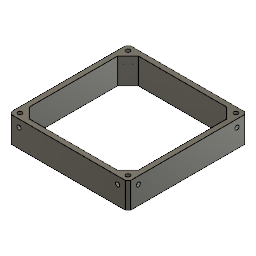
stucture lower fossasat v2 (Autodesk Fusion 360 design; units mm, degrees)
Autodesk Fusion 360 part; units mm, degrees
note: some values were not read from the file. Set by a fixed rule: which sketch regions a step uses.
sketch "Sketch1" plane through (0, 0, 0) normal (0, 1, 0) x (1, 0, 0)
  line L0 (0, 0) -> (46, 0)
  line L1 (46, 0) -> (46, -46)
  line L2 (46, -46) -> (0, -46)
  line L3 (0, -46) -> (0, 0)
  line L4 (0, 0) -> (6.364, -6.364)
  line L5 (0, 0) -> (9, 0) construction
  line L6 (6.364, -6.364) -> (0, -6.364)
  line L7 (0, -6.364) -> (0, 0)
  line L8 (0, 0) -> (6.364, 0)
  line L9 (6.364, 0) -> (6.364, -6.364)
  line L10 (46, -46) -> (37, -46)
  line L11 (37, -46) -> (37, -37)
  line L12 (37, -37) -> (46, -37)
  line L13 (46, -37) -> (46, -46)
  line L14 (46, 0) -> (37, 0)
  line L15 (37, 0) -> (37, -9)
  line L16 (37, -9) -> (46, -9)
  line L17 (46, -9) -> (46, 0)
  line L18 (0, -46) -> (9, -46)
  line L19 (9, -46) -> (9, -37)
  line L20 (9, -37) -> (0, -37)
  line L21 (0, -37) -> (0, -46)
  line L22 (0, -46) -> (2, -46)
  line L23 (2, -46) -> (2, -44)
  circle A0 centre (2, -44) radius 1
  circle A1 centre (2, -44) radius 0.8
  line L24 (23, 0) -> (23, -46)
  line L25 (23, -23) -> (42, -23)
  line L26 (42, -23) -> (42, -42)
  line L27 (42, -42) -> (4, -42)
  line L28 (4, -42) -> (4, -4)
  line L29 (4, -4) -> (42, -4)
  line L30 (42, -4) -> (42, -42)
  line L31 (4, -42) -> (8, -46)
  line L32 (4, -42) -> (9.6569, -42) construction
  line L33 (8, -46) -> (0, -38)
  line L34 (46, -46) -> (44, -46)
  line L35 (44, -46) -> (44, -44)
  circle A2 centre (44, -44) radius 0.8
  line L36 (42, -42) -> (46, -38)
  line L37 (42, -42) -> (38, -46)
  line L38 (46, 0) -> (44, 0)
  line L39 (44, 0) -> (44, -2)
  circle A3 centre (44, -2) radius 0.8
  line L40 (42, -4) -> (46, -8)
  line L41 (46, -8) -> (38, 0)
  line L42 (4, -4) -> (8, 0)
  line L43 (4, -4) -> (0, -8)
  line L44 (0, 0) -> (1.4142, -1.4142)
  circle A4 centre (1.4142, -1.4142) radius 0.8
  line L45 (23, 0) -> (23, -2)
  line L46 (40, -2) -> (6, -2)
  line L47 (44, -6) -> (44, -40)
  line L48 (40, -44) -> (6, -44)
  line L49 (2, -40) -> (2, -6)
  dimension "d1" = 46
  dimension "d2" = 46
  dimension "d3" = 45
  dimension "d4" = 9
  dimension "d5" = 9
  dimension "d6" = 9
  dimension "d7" = 9
  dimension "d8" = 9
  dimension "d9" = 9
  dimension "d10" = 2
  dimension "d11" = 1.6
  dimension "d12" = 19
  dimension "d13" = 19
  dimension "d14" = 45
  dimension "d15" = 1.6
  measures "d3" angle of L4 L5
  measures "d4" distance of L0.start
  measures "d8" distance of L0.start
  measures "d10" distance of L0.start
  measures "d11" diameter of A1
  measures "d14" angle of L31 L32
  measures "d15" diameter of A2
extrude "Extrude1" add sketch "Sketch1" along normal blind 10 contours L3 L4 L6 L7 L43 L44 A4 | L0 L4 L8 L9 L42 L44 A4 | L0 L9 L42 | L3 L6 L43 | L0 L9 L24 L42 L45 L46 | L9 L42 L46 | L3 L6 L20 L43 L49 | L0 L15 L24 L45 L46 | L3 L20 L21 L33 L49 | L0 L14 L15 L41 L46 | L2 L3 L18 L21 L22 L31 L33 | L0 L1 L14 L17 L38 L40 L41 | L2 L18 L19 L31 L33 L48 | L1 L16 L17 L40 L41 L47 | L2 L11 L24 L48 | L2 L19 L24 L48 | L1 L12 L16 L47 | L2 L10 L11 L37 L48 | L1 L2 L10 L13 L34 L36 L37 | L1 L12 L13 L36 L47
sketch "Sketch2" plane through (46, 0, 0) normal (1, 0, 0) x (0, 0, -1)
  line L0 (-46, 0) -> (0, 0)
  line L1 (0, 0) -> (0, 10)
  line L2 (0, 10) -> (-46, 10)
  line L3 (-46, 10) -> (-46, 0)
  line L4 (-43, 0) -> (-43, 7.15)
  line L5 (-43, 7.15) -> (-46.6287, 7.15)
  line L6 (-46, 7.15) -> (-42, 7.15)
  circle A0 centre (-42, 7.15) radius 0.8
extrude "Extrude2" cut sketch "Sketch2" against normal blind 3 contours A0
sketch "Sketch3" plane through (0, 0, 46) normal (0, 0, 1) x (1, 0, 0)
  line L0 (0, 0) -> (46, 0)
  line L1 (46, 0) -> (46, 10)
  line L2 (46, 10) -> (0, 10)
  line L3 (0, 10) -> (0, 0)
  line L4 (43.2, 0) -> (43.2, 7.15)
  line L5 (43.2, 7.15) -> (46.5827, 7.15)
  line L6 (46, 7.15) -> (42, 7.15)
  circle A0 centre (42, 7.15) radius 0.8
  dimension "d20" = 7.15
  dimension "d21" = 1.6
  measures "d20" distance of L0.start
  measures "d21" diameter of A0
extrude "Extrude3" cut sketch "Sketch3" against normal blind 3 contours A0
sketch "Sketch4" plane through (46, 0, 0) normal (1, 0, 0) x (0, 0, -1)
  circle A0 centre (-42, 7.15) radius 0.8
  line L0 (-46, 0) -> (0, 0)
  line L1 (0, 0) -> (0, 10)
  line L2 (0, 10) -> (-46, 10)
  line L3 (-46, 10) -> (-46, 0)
  line L4 (0, 0) -> (-4, 0)
  line L5 (-4, 0) -> (-4, 7.15)
  circle A1 centre (-4, 7.15) radius 0.8
extrude "Extrude4" cut sketch "Sketch4" against normal blind 3 contours A1
sketch "Sketch5" plane through (0, 0, 0) normal (0, 0, -1) x (-1, 0, 0)
  line L0 (-46, 0) -> (0, 0)
  line L1 (0, 0) -> (0, 10)
  line L2 (0, 10) -> (-46, 10)
  line L3 (-46, 10) -> (-46, 0)
  line L4 (-46, 0) -> (-42, 0)
  line L5 (-42, 0) -> (-42, 7.15)
  circle A0 centre (-42, 7.15) radius 0.8
extrude "Extrude5" cut sketch "Sketch5" against normal blind 3 contours A0
sketch "Sketch6" plane through (0, 0, 0) normal (0, 0, -1) x (-1, 0, 0)
  circle A0 centre (-42, 7.15) radius 0.8
  line L0 (-46, 0) -> (0, 0)
  line L1 (0, 0) -> (0, 10)
  line L2 (0, 10) -> (-46, 10)
  line L3 (-46, 10) -> (-46, 0)
  line L4 (0, 0) -> (-4, 0)
  line L5 (-4, 0) -> (-4, 7.15)
  circle A1 centre (-4, 7.15) radius 0.8
extrude "Extrude6" cut sketch "Sketch6" against normal blind 3 contours A1
sketch "Sketch7" plane through (0, 0, 0) normal (-1, 0, 0) x (0, 0, 1)
  line L0 (0, 0) -> (46, 0)
  line L1 (46, 0) -> (46, 10)
  line L2 (46, 10) -> (0, 10)
  line L3 (0, 10) -> (0, 0)
  line L4 (0, 0) -> (4, 0)
  line L5 (4, 0) -> (4, 7.15)
  line L6 (46, 0) -> (42, 0)
  line L7 (42, 0) -> (42, 7.15)
  circle A0 centre (42, 7.15) radius 0.8
  circle A1 centre (4, 7.15) radius 0.8
extrude "Extrude7" cut sketch "Sketch7" against normal blind 3 contours A0 | A1
sketch "Sketch8" plane through (0, 10, 0) normal (0, 1, 0) x (-1, 0, 0)
  circle A0 centre (-1.4142, 1.4142) radius 0.8
  circle A1 centre (-44, 2) radius 0.8
  line L0 (-44, 40) -> (-42, 42)
  line L1 (-42, 42) -> (-40, 44)
  line L2 (-40, 44) -> (-6, 44)
  line L3 (-6, 44) -> (-2, 40)
  line L4 (-2, 40) -> (-2, 6.364)
  line L5 (-2, 6.364) -> (-1.636, 6.364)
  line L6 (-1.636, 6.364) -> (-6, 2)
  line L7 (-6, 2) -> (-40, 2)
  line L8 (-40, 2) -> (-44, 6)
  line L9 (-44, 6) -> (-44, 40)
  circle A2 centre (-44, 44) radius 0.8
  circle A3 centre (-2, 44) radius 1
  line L10 (-46, 46) -> (-46, 0)
  line L11 (-46, 0) -> (0, 0)
  line L12 (0, 0) -> (0, 46)
  line L13 (0, 46) -> (-46, 46)
  circle A4 centre (-2, 44) radius 1
  circle A5 centre (-2, 44) radius 0.8
extrude "Extrude8" add sketch "Sketch8" against normal blind 10 contours A3 A4
sketch "Sketch9" plane through (0, 0, 46) normal (0, 0, 1) x (1, 0, 0)
  circle A0 centre (42, 7.15) radius 0.8
  line L0 (0, 0) -> (46, 0)
  line L1 (46, 0) -> (46, 10)
  line L2 (46, 10) -> (0, 10)
  line L3 (0, 10) -> (0, 0)
  line L4 (0, 0) -> (4, 0)
  line L5 (4, 0) -> (4, 7.15)
  circle A1 centre (4, 7.15) radius 0.8
extrude "Extrude9" cut sketch "Sketch9" against normal blind 3 contours A1
sketch "Sketch10" plane through (0, 10, 0) normal (0, 1, 0) x (-1, 0, 0)
  circle A0 centre (-2, 44) radius 0.8
  circle A1 centre (-1.4142, 1.4142) radius 0.8
  circle A2 centre (-44, 2) radius 0.8
  line L0 (-44, 40) -> (-42, 42)
  line L1 (-42, 42) -> (-40, 44)
  line L2 (-40, 44) -> (-6, 44)
  line L3 (-6, 44) -> (-2, 40)
  line L4 (-2, 40) -> (-2, 6.364)
  line L5 (-2, 6.364) -> (-1.636, 6.364)
  line L6 (-1.636, 6.364) -> (-6, 2)
  line L7 (-6, 2) -> (-40, 2)
  line L8 (-40, 2) -> (-44, 6)
  line L9 (-44, 6) -> (-44, 40)
  circle A3 centre (-44, 44) radius 0.8
  line L10 (-46, 46) -> (-46, 0)
  line L11 (-46, 0) -> (0, 0)
  line L12 (0, 0) -> (0, 46)
  line L13 (0, 46) -> (-46, 46)
  line L14 (-2, 6.364) -> (-2, 5.5)
  line L15 (-2, 5.5) -> (-1.568, 5.932)
  line L16 (-1.568, 5.932) -> (-1.5, 7)
  line L17 (-1.5, 7) -> (-2, 6.364)
extrude "Extrude10" add sketch "Sketch10" against normal blind 10 contours L5 L6 L14
sketch "Sketch11" plane through (0, 10, 0) normal (0, 1, 0) x (-1, 0, 0)
  circle A0 centre (-2, 44) radius 0.8
  circle A1 centre (-1.4142, 1.4142) radius 0.8
  circle A2 centre (-44, 2) radius 0.8
  line L0 (-44, 40) -> (-42, 42)
  line L1 (-42, 42) -> (-40, 44)
  line L2 (-40, 44) -> (-6, 44)
  line L3 (-6, 44) -> (-2, 40)
  line L4 (-2, 40) -> (-2, 6)
  line L5 (-2, 6) -> (-6, 2)
  line L6 (-6, 2) -> (-40, 2)
  line L7 (-40, 2) -> (-44, 6)
  line L8 (-44, 6) -> (-44, 40)
  circle A3 centre (-44, 44) radius 0.8
  line L9 (-46, 46) -> (-46, 0)
  line L10 (-46, 0) -> (0, 0)
  line L11 (0, 0) -> (0, 46)
  line L12 (0, 46) -> (-46, 46)
  circle A4 centre (-1.4142, 1.4142) radius 0.8
extrude "Extrude11" add sketch "Sketch11" against normal blind 10 contours A1 A4
sketch "Sketch12" plane through (0, 10, 0) normal (0, 1, 0) x (-1, 0, 0)
  circle A0 centre (-2, 44) radius 0.8
  circle A1 centre (-44, 2) radius 0.8
  line L0 (-44, 40) -> (-42, 42)
  line L1 (-42, 42) -> (-40, 44)
  line L2 (-40, 44) -> (-6, 44)
  line L3 (-6, 44) -> (-2, 40)
  line L4 (-2, 40) -> (-2, 6)
  line L5 (-2, 6) -> (-6, 2)
  line L6 (-6, 2) -> (-40, 2)
  line L7 (-40, 2) -> (-44, 6)
  line L8 (-44, 6) -> (-44, 40)
  circle A2 centre (-44, 44) radius 0.8
  line L9 (-46, 46) -> (-46, 0)
  line L10 (-46, 0) -> (0, 0)
  line L11 (0, 0) -> (0, 46)
  line L12 (0, 46) -> (-46, 46)
  line L13 (0, 0) -> (-2, 0)
  line L14 (-2, 0) -> (-2, 2)
  circle A3 centre (-2, 2) radius 0.8
extrude "Extrude12" cut sketch "Sketch12" against normal blind 24.5 contours A3
chamfer "Chamfer1" distance 1 angle 45 4 edges at (0, 5, 0) (0, 5, 46) (46, 5, 46) (46, 5, 0)
sketch "Sketch13" plane through (0, 10, 0) normal (0, 1, 0) x (-1, 0, 0)
  line L0 (-46, 1) -> (-45, 0)
  line L1 (-45, 0) -> (-1, 0)
  line L2 (-1, 0) -> (0, 1)
  line L3 (0, 1) -> (0, 45)
  line L4 (0, 45) -> (-1, 46)
  line L5 (-1, 46) -> (-45, 46)
  line L6 (-45, 46) -> (-46, 45)
  line L7 (-46, 45) -> (-46, 1)
  circle A0 centre (-2, 2) radius 0.8
  circle A1 centre (-2, 44) radius 0.8
  circle A2 centre (-44, 2) radius 0.8
  line L8 (-44, 40) -> (-42, 42)
  line L9 (-42, 42) -> (-40, 44)
  line L10 (-40, 44) -> (-6, 44)
  line L11 (-6, 44) -> (-2, 40)
  line L12 (-2, 40) -> (-2, 6)
  line L13 (-2, 6) -> (-6, 2)
  line L14 (-6, 2) -> (-40, 2)
  line L15 (-40, 2) -> (-44, 6)
  line L16 (-44, 6) -> (-44, 40)
  circle A3 centre (-44, 44) radius 0.8
extrude "Extrude13" add sketch "Sketch13" against normal blind 10 contours A0 | A1 | A2 | A3
sketch "Sketch14" plane through (0, 10, 0) normal (0, 1, 0) x (-1, 0, 0)
  line L0 (-46, 1) -> (-45, 0)
  line L1 (-45, 0) -> (-1, 0)
  line L2 (-1, 0) -> (0, 1)
  line L3 (0, 1) -> (0, 45)
  line L4 (0, 45) -> (-1, 46)
  line L5 (-1, 46) -> (-45, 46)
  line L6 (-45, 46) -> (-46, 45)
  line L7 (-46, 45) -> (-46, 1)
  line L8 (-44, 40) -> (-42, 42)
  line L9 (-42, 42) -> (-40, 44)
  line L10 (-40, 44) -> (-6, 44)
  line L11 (-6, 44) -> (-2, 40)
  line L12 (-2, 40) -> (-2, 6)
  line L13 (-2, 6) -> (-6, 2)
  line L14 (-6, 2) -> (-40, 2)
  line L15 (-40, 2) -> (-44, 6)
  line L16 (-44, 6) -> (-44, 40)
  line L17 (0, 0) -> (-2.2, 0)
  line L18 (-2.2, 0) -> (-2.2, 2.2)
  line L19 (-46, 0) -> (-46, 2.2)
  line L20 (-46, 2.2) -> (-43.8, 2.2)
  line L21 (-46, 46) -> (-46, 43.8)
  line L22 (-46, 43.8) -> (-43.8, 43.8)
  line L23 (0, 46) -> (-2.2, 46)
  line L24 (-2.2, 46) -> (-2.2, 43.8)
  circle A0 centre (-2.2, 43.8) radius 0.8
  circle A1 centre (-43.8, 43.8) radius 0.8
  circle A2 centre (-43.8, 2.2) radius 0.8
  circle A3 centre (-2.2, 2.2) radius 0.8
  dimension "d46" = 2.2
  dimension "d47" = 1.6
  measures "d47" diameter of A2
extrude "Extrude14" cut sketch "Sketch14" against normal blind 20 contours A0 | A1 | A2 | A3
